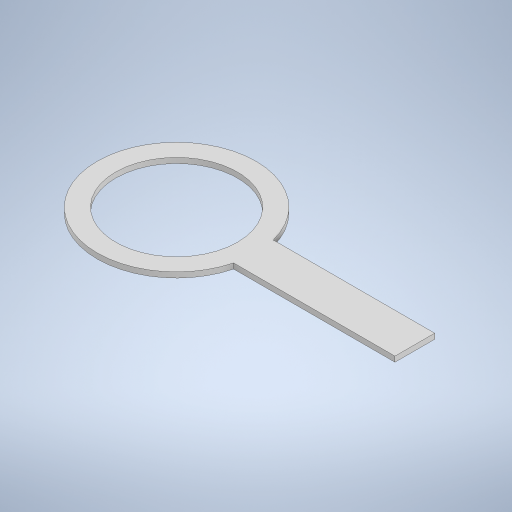
# Autodesk Inventor part: 압력센서
Saved by Autodesk Inventor 2024 (Build 280153000, 153)
## iProperties
Created: 2024-04-21
Part Number: 압력센서
Material: 일반
Document SubType Name: Modeling
Designer: kkamin5
Density: 1 g/cm^3
Appearance: 기본값
Author: kkamin5
Autodesk Inventor part; units mm, degrees
ref_plane "YZ Plane" through (0, 0, 0) normal (1, 0, 0) x (0, 1, 0)
ref_plane "XZ Plane" through (0, 0, 0) normal (0, 1, 0) x (-1, 0, 0)
ref_plane "XY Plane" through (0, 0, 0) normal (0, 0, 1) x (1, 0, 0)
sketch "스케치1" plane through (0, 0, 0) normal (0, 1, 0) x (-1, 0, 0)
  circle A0 centre (0, 0) radius 15
  circle A1 centre (0, 0) radius 11.5
  line L0 (-14.5237, 3.75) -> (-45, 3.75)
  line L1 (-45, 3.75) -> (-45, -3.75)
  line L2 (-45, -3.75) -> (-14.5237, -3.75)
  line L3 (-14.5237, -3.75) -> (-14.5237, 3.75)
  dimension "d0" = 30
  dimension "d1" = 23
  dimension "d2" = 7.5
  dimension "d3" = 3.75
  dimension "d4" = 45
  constraints: 8 end point, 2 coincident, 2 parallel, 1 centre point, 1 horizontal, 1 perpendicular, 3 other
  measures "d1" diameter of A1
  measures "d2" distance of L0.end L1.end
  measures "d3" distance from line of point (0, 0) L2
  measures "d4" horizontal distance of point (0, 0) L0.end
extrude "돌출1" add sketch "스케치1" along normal blind 1
